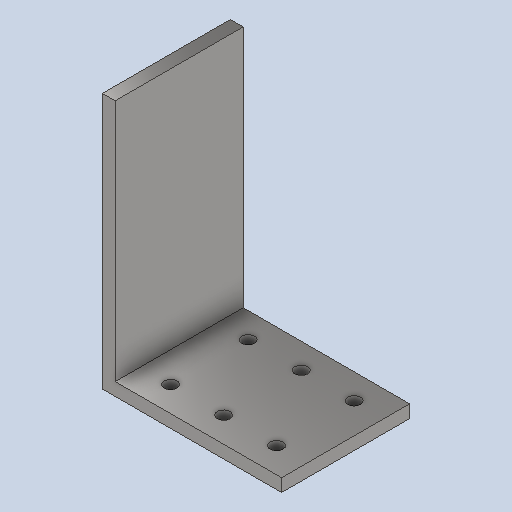
# Autodesk Inventor part: L_Channel
Saved by Autodesk Inventor 2023 (Build 270158000, 158)
## iProperties
Created: 2025-04-19
Part Number: L_Channel
Material: Steel, Mild
Document SubType Name: Modeling
Designer: plebbb
Density: 7.85 g/cm^3
Appearance: Semi-Polished
Author: plebbb
Autodesk Inventor part; units mm, degrees
ref_plane "YZ Plane" through (0, 0, 0) normal (1, 0, 0) x (0, 1, 0)
ref_plane "XZ Plane" through (0, 0, 0) normal (0, 1, 0) x (-1, 0, 0)
ref_plane "XY Plane" through (0, 0, 0) normal (0, 0, 1) x (1, 0, 0)
sketch "Sketch1" plane through (0, 0, 0) normal (0, 0, 1) x (1, 0, 0)
  line L0 (0, 0) -> (88.9, 0)
  line L1 (88.9, 0) -> (88.9, 6.35)
  line L2 (88.9, 6.35) -> (6.35, 6.35)
  line L3 (6.35, 6.35) -> (6.35, 44.45)
  line L4 (6.35, 44.45) -> (6.35, 127)
  line L5 (6.35, 127) -> (0, 127)
  line L6 (0, 127) -> (0, 0)
  dimension "d0" = 88.9
  dimension "d1" = 127
  dimension "d2" = 6.35
  constraints: 14 end point, 6 perpendicular, 1 horizontal, 1 point on line
  measures "d0" distance of L0.start L0.end
  measures "d1" distance of L5.end L0.start
  measures "d2" distance of L4.end L5.end
extrude "Extrusion1" add sketch "Sketch1" along normal blind 63.5
sketch "Sketch2" plane through (6.35, 6.35, 0) normal (0, 1, 0) x (1, 0, 0)
  line L0 (67.55, -51) -> (15, -51) construction
  line L1 (15, -51) -> (15, -12.5) construction
  line L2 (15, -12.5) -> (67.55, -12.5) construction
  line L3 (67.55, -12.5) -> (67.55, -51) construction
  circle A0 centre (67.55, -51) radius 3.175
  circle A1 centre (67.55, -12.5) radius 3.175
  circle A2 centre (41.275, -51) radius 3.175
  circle A3 centre (41.275, -12.5) radius 3.175
  circle A4 centre (15, -51) radius 3.175
  circle A5 centre (15, -12.5) radius 3.175
  line L4 (0, 0) -> (82.55, 0) construction
  line L5 (82.55, 0) -> (82.55, -63.5) construction
  line L6 (82.55, -63.5) -> (0, -63.5) construction
  line L7 (0, -63.5) -> (0, 0) construction
  line L8 (67.55, -31.75) -> (82.55, -31.75) construction
  line L9 (15, -31.75) -> (0, -31.75) construction
  point P0 (-6.35, 0)
  dimension "d5" = 6.35
  dimension "d6" = 6.35
  dimension "d7" = 63.5
  dimension "d9" = 88.9
  dimension "d10" = 15
  dimension "d11" = 12.5
  constraints: 20 end point, 6 centre point, 6 midpoint, 5 equal radius, 4 coincident, 4 parallel, 3 horizontal, 2 perpendicular, 1 collinear, 1 horizontal alignment
  measures "d5" diameter of A0
  measures "d6" distance of point (-6.35, 0) L4.start
  measures "d7" distance of L6.end L4.start
  measures "d9" horizontal distance of L5.end point (-6.35, 0)
  measures "d10" distance of L8.start L8.end
  measures "d11" distance from line of L6 A2.centre
extrude "Extrusion2" cut sketch "Sketch2" against normal through all
body "Solid1"
